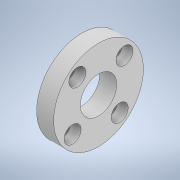
# Autodesk Inventor part: MotorMount
Saved by Autodesk Inventor 2022 (Build 260153000, 153)
## iProperties
Created: 2022-02-05
Part Number: MotorMount
Material: Generic
Document SubType Name: Modeling
Designer: ultra
Density: 1 g/cm^3
Appearance: Default
Author: ultra
Autodesk Inventor part; units mm, degrees
ref_plane "YZ Plane" through (0, 0, 0) normal (1, 0, 0) x (0, 1, 0)
ref_plane "XZ Plane" through (0, 0, 0) normal (0, 1, 0) x (-1, 0, 0)
ref_plane "XY Plane" through (0, 0, 0) normal (0, 0, 1) x (1, 0, 0)
sketch "Sketch1" plane through (0, 0, 0) normal (1, 0, 0) x (0, 1, 0)
  arc A0 (-16.1342, -4.5) -> (-16.1342, 4.5) centre (0, 0) ccw
  line L0 (-10.6472, 4.5) -> (-16.1342, 4.5)
  line L1 (-10.6472, -4.5) -> (-10.6472, 4.5)
  line L2 (-16.1342, -4.5) -> (-10.6472, -4.5)
  circle A1 centre (9.6916, 7.8945) radius 1.5
  circle A2 centre (7.8945, -9.6916) radius 1.5
  circle A3 centre (-9.6916, -7.8945) radius 1.5
  circle A4 centre (-7.8945, 9.6916) radius 1.5
  circle A5 centre (0, 0) radius 6.8
  circle A6 centre (9.6916, 7.8945) radius 1.5875
  circle A7 centre (7.8945, -9.6916) radius 1.5875
  circle A8 centre (-9.6916, -7.8945) radius 1.5875
  circle A9 centre (-7.8945, 9.6916) radius 1.5875
  circle A10 centre (0, 0) radius 16.75
  point P0 (-16.1342, -4.5)
  point P1 (-16.1342, 4.5)
  dimension "d2" = 3.175
  dimension "d3" = 3.175
  dimension "d4" = 3.175
  dimension "d5" = 3.175
  constraints: 11 centre point, 6 end point, 5 coincident, 2 point on circle, 1 concentric
  measures "d2" diameter of A6
  measures "d3" diameter of A7
  measures "d4" diameter of A8
  measures "d5" diameter of A9
extrude "Extrusion3" add sketch "Sketch1" along normal blind 6.35 contours L2 L1 L0 A0 | A10 L0 L1 L2
sketch "Sketch3" plane through (6.35, 0, 0) normal (1, 0, 0) x (0, 0, -1)
  circle A0 centre (-9.6916, -7.8945) radius 1.5875 projected
  circle A1 centre (7.8945, -9.6916) radius 1.5875 projected
  circle A2 centre (9.6916, 7.8945) radius 1.5875 projected
  circle A3 centre (-7.8945, 9.6916) radius 1.5875 projected
  circle A4 centre (-7.8945, 9.6916) radius 3.175
  circle A5 centre (9.6916, 7.8945) radius 3.175
  circle A6 centre (7.8945, -9.6916) radius 3.175
  circle A7 centre (-9.6916, -7.8945) radius 3.175
  dimension "d14" = 6.35
  dimension "d15" = 6.35
  dimension "d16" = 6.35
  dimension "d17" = 6.35
  constraints: 4 centre point, 4 coincident
  measures "d14" diameter of A4
  measures "d15" diameter of A5
  measures "d16" diameter of A6
  measures "d17" diameter of A7
extrude "Extrusion4" cut sketch "Sketch3" against normal blind 4
body "Solid3"
